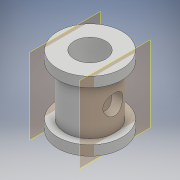
# Autodesk Inventor part: firstSpindle
Saved by Autodesk Inventor 2018 (Build 220112000, 112)
## iProperties
Created: 2017-10-12
Part Number: firstSpindle
Material: Generic
Document SubType Name: Modeling
Designer: Payal Jindal
Density: 1 g/cm^3
Appearance: Default
Author: Payal Jindal
Autodesk Inventor part; units mm, degrees
ref_plane "XZ Plane" through (0, 0, 0) normal (0, 1, 0) x (-1, 0, 0)
ref_plane "XY Plane" through (0, 0, 0) normal (0, 0, 1) x (1, 0, 0)
sketch "Sketch1" plane through (0, 0, 0) normal (0, 0, 1) x (1, 0, 0)
  circle A0 centre (0, 0) radius 5
  circle A1 centre (0, 0) radius 3.175
  dimension "d0" = 10
  dimension "d1" = 6.35
  constraints: 2 centre point, 2 coincident
  measures "d0" diameter of A0
  measures "d1" diameter of A1
extrude "Extrusion1" add sketch "Sketch1" along normal blind 10
sketch "Sketch2" plane through (0, 0, 10) normal (0, 0, 1) x (1, 0, 0)
  circle A0 centre (0, 0) radius 6.5
  circle A1 centre (0, 0) radius 3.175 projected
  dimension "d4" = 13
  constraints: 1 centre point, 1 coincident
  measures "d4" diameter of A0
sketch "Sketch4" plane through (0, 0, 0) normal (0, 0, -1) x (-1, 0, 0)
  circle A0 centre (0, 0) radius 6.5
  circle A1 centre (0, 0) radius 3.175 projected
  dimension "d8" = 13
  constraints: 1 centre point, 1 coincident
  measures "d8" diameter of A0
extrude "Extrusion4" add sketch "Sketch2" along normal blind 2
extrude "Extrusion5" add sketch "Sketch4" along normal blind 2
ref_plane "Work Plane1" through (5, 0, 0) normal (1, 0, 0) x (0, 1, 0)
sketch "Sketch5" plane through (5, 0, 0) normal (1, 0, 0) x (0, 1, 0)
  line L0 (6.5, 0) -> (-6.5, 0) projected
  line L1 (-6.5, 10) -> (6.5, 10) projected
  line L2 (0, 0) -> (0, 10)
  point P0 (0, 5)
  constraints: 2 end point, 2 midpoint
hole "Hole1" at (5, 0, 5) direction (-1, 0, 0) diameter 3 end through all counterbore diameter 4 counterbore depth 3
ref_plane "Work Plane2" through (-5, 0, 0) normal (1, 0, 0) x (0, 1, 0)
sketch "Sketch6" plane through (-5, 0, 0) normal (1, 0, 0) x (0, 1, 0)
  line L0 (0, 3.5) -> (0, 3.5)
  point P0 (0, 0)
  point P1 (1.5, 5)
  constraints: 2 end point, 1 vertical, 3 other
equation "\"d13\" = lip"
equation "\"d15\" = lip"
equation "\"lip\" = 2"
body "Solid1"
